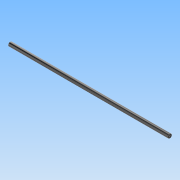
# Autodesk Inventor part: вал 8мм ось x
Saved by Autodesk Inventor 2017 (Build 210142000, 142)
## iProperties
Part Number: вал 8мм ось x
Material: Типовые
Document SubType Name: Modeling
Designer: Max
Mass: 15.3626 g
Surface Area: 79.7684 cm^2
Volume: 15.3626 cm^3
Density: 1 g/cm^3
Appearance: Сталь — полированная
Author: Max
Autodesk Inventor part; units mm, degrees
ref_plane "YZ Plane" through (0, 0, 0) normal (1, 0, 0) x (0, 1, 0)
ref_plane "XZ Plane" through (0, 0, 0) normal (0, 1, 0) x (-1, 0, 0)
ref_plane "XY Plane" through (0, 0, 0) normal (0, 0, 1) x (1, 0, 0)
sketch "Эскиз1" plane through (0, 0, 0) normal (1, 0, 0) x (0, 1, 0)
  circle A0 centre (0, 0) radius 4
  circle A1 centre (0, 0) radius 1.5
  dimension "d0" = 8
  dimension "d1" = 3
  constraints: 2 centre point, 2 coincident
  measures "d0" diameter of A0
  measures "d1" diameter of A1
extrude "Выдавливание1" add sketch "Эскиз1" along normal mid plane 308 contours A0 | A1
sketch "Эскиз2" plane through (154, 0, 0) normal (1, 0, 0) x (0, 0, -1)
  circle A0 centre (0, 0) radius 1.5
  dimension "d4" = 3
  constraints: 1 centre point, 1 coincident
  measures "d4" diameter of A0
extrude "Выдавливание2" cut sketch "Эскиз2" against normal blind 8
sketch "Эскиз3" plane through (-154, 0, 0) normal (-1, 0, 0) x (0, 0, 1)
  circle A0 centre (0, 0) radius 1.5
  dimension "d7" = 3
  constraints: 1 centre point, 1 coincident
  measures "d7" diameter of A0
extrude "Выдавливание3" cut sketch "Эскиз3" against normal blind 8
chamfer "Фаска1" distance 0.5 angle 45 2 edges at (-154, -4, 0) (154, -4, 0)
